Autodesk Inventor part; units mm, degrees
(part 3 of 3)
  line L1297 (279.9003, 88.0576) -> (279.8208, 87.9559)
  line L1298 (279.8208, 87.9559) -> (279.7345, 87.86)
  line L1299 (279.7345, 87.86) -> (279.6416, 87.7704)
  line L1300 (279.6416, 87.7704) -> (279.5428, 87.6874)
  line L1301 (279.5428, 87.6874) -> (279.4383, 87.6115)
  line L1302 (279.4383, 87.6115) -> (279.3289, 87.5431)
  line L1303 (279.3289, 87.5431) -> (279.2149, 87.4825)
  line L1304 (279.2149, 87.4825) -> (279.097, 87.43)
  line L1305 (279.097, 87.43) -> (278.9757, 87.3859)
  line L1306 (278.9757, 87.3859) -> (278.8517, 87.3503)
  line L1307 (278.8517, 87.3503) -> (278.7254, 87.3235)
  line L1308 (278.7254, 87.3235) -> (278.5976, 87.3055)
  line L1309 (278.5976, 87.3055) -> (278.4689, 87.2965)
  line L1310 (278.4689, 87.2965) -> (278.3398, 87.2965)
  line L1311 (278.3398, 87.2965) -> (278.211, 87.3055)
  line L1312 (278.211, 87.3055) -> (278.0832, 87.3235)
  line L1313 (278.0832, 87.3235) -> (277.957, 87.3503)
  line L1314 (277.957, 87.3503) -> (277.8329, 87.3859)
  line L1315 (277.8329, 87.3859) -> (277.7116, 87.43)
  line L1316 (277.7116, 87.43) -> (277.5937, 87.4825)
  line L1317 (277.5937, 87.4825) -> (277.4798, 87.5431)
  line L1318 (277.4798, 87.5431) -> (277.3703, 87.6115)
  line L1319 (277.3703, 87.6115) -> (277.2659, 87.6874)
  line L1320 (277.2659, 87.6874) -> (277.167, 87.7704)
  line L1321 (277.167, 87.7704) -> (277.0742, 87.86)
  line L1322 (277.0742, 87.86) -> (276.9878, 87.9559)
  line L1323 (276.9878, 87.9559) -> (276.9084, 88.0576)
  line L1324 (276.9084, 88.0576) -> (276.8362, 88.1646)
  line L1325 (276.8362, 88.1646) -> (276.7716, 88.2764)
  line L1326 (276.7716, 88.2764) -> (276.7151, 88.3924)
  line L1327 (276.7151, 88.3924) -> (276.6667, 88.5121)
  line L1328 (276.6667, 88.5121) -> (276.6268, 88.6348)
  line L1329 (276.6268, 88.6348) -> (276.5956, 88.7601)
  line L1330 (276.5956, 88.7601) -> (276.5732, 88.8872)
  line L1331 (276.5732, 88.8872) -> (276.5597, 89.0155)
  line L1332 (276.5597, 89.0155) -> (276.5552, 89.1445)
  line L1333 (276.5552, 89.1445) -> (276.5597, 89.2735)
  line L1334 (276.5597, 89.2735) -> (276.5732, 89.4019)
  line L1335 (276.5732, 89.4019) -> (276.5956, 89.529)
  line L1336 (276.5956, 89.529) -> (276.6268, 89.6542)
  line L1337 (276.6268, 89.6542) -> (276.6667, 89.777)
  line L1338 (276.6667, 89.777) -> (276.7151, 89.8966)
  line L1339 (276.7151, 89.8966) -> (276.7716, 90.0126)
  line L1340 (276.7716, 90.0126) -> (276.8362, 90.1244)
  line L1341 (276.8362, 90.1244) -> (276.9084, 90.2314)
  line L1342 (276.9084, 90.2314) -> (276.9878, 90.3331)
  line L1343 (276.9878, 90.3331) -> (277.0742, 90.429)
  line L1344 (277.0742, 90.429) -> (277.167, 90.5187)
  line L1345 (277.167, 90.5187) -> (277.2659, 90.6016)
  line L1346 (277.2659, 90.6016) -> (277.3703, 90.6775)
  line L1347 (277.3703, 90.6775) -> (277.4798, 90.7459)
  line L1348 (277.4798, 90.7459) -> (277.5937, 90.8065)
  line L1349 (277.5937, 90.8065) -> (277.7116, 90.859)
  line L1350 (277.7116, 90.859) -> (277.8329, 90.9031)
  line L1351 (277.8329, 90.9031) -> (277.957, 90.9387)
  line L1352 (277.957, 90.9387) -> (278.0832, 90.9655)
  line L1353 (278.0832, 90.9655) -> (278.211, 90.9835)
  line L1354 (278.211, 90.9835) -> (278.3398, 90.9925)
  line L1355 (278.3398, 90.9925) -> (278.4689, 90.9925)
  line L1356 (278.4689, 90.9925) -> (278.5976, 90.9835)
  line L1357 (278.5976, 90.9835) -> (278.7254, 90.9655)
  line L1358 (278.7254, 90.9655) -> (278.8517, 90.9387)
  line L1359 (278.8517, 90.9387) -> (278.9757, 90.9031)
  line L1360 (278.9757, 90.9031) -> (279.097, 90.859)
  line L1361 (279.097, 90.859) -> (279.2149, 90.8065)
  line L1362 (279.2149, 90.8065) -> (279.3289, 90.7459)
  line L1363 (279.3289, 90.7459) -> (279.4383, 90.6775)
  line L1364 (279.4383, 90.6775) -> (279.5428, 90.6016)
  line L1365 (279.5428, 90.6016) -> (279.6416, 90.5187)
  line L1366 (279.6416, 90.5187) -> (279.7345, 90.429)
  line L1367 (279.7345, 90.429) -> (279.8208, 90.3331)
  line L1368 (279.8208, 90.3331) -> (279.9003, 90.2314)
  line L1369 (279.9003, 90.2314) -> (279.9725, 90.1244)
  line L1370 (279.9725, 90.1244) -> (280.037, 90.0126)
  line L1371 (280.037, 90.0126) -> (280.0936, 89.8966)
  line L1372 (280.0936, 89.8966) -> (280.1419, 89.777)
  line L1373 (280.1419, 89.777) -> (280.1818, 89.6542)
  line L1374 (280.1818, 89.6542) -> (280.213, 89.529)
  line L1375 (280.213, 89.529) -> (280.2354, 89.4019)
  line L1376 (280.2354, 89.4019) -> (280.2489, 89.2735)
  line L1377 (280.2489, 89.2735) -> (280.2534, 89.1445)
  line L1378 (280.2534, 17.1431) -> (280.2489, 17.0142)
  line L1379 (280.2489, 17.0142) -> (280.2354, 16.8858)
  line L1380 (280.2354, 16.8858) -> (280.213, 16.7587)
  line L1381 (280.213, 16.7587) -> (280.1818, 16.6335)
  line L1382 (280.1818, 16.6335) -> (280.1419, 16.5107)
  line L1383 (280.1419, 16.5107) -> (280.0936, 16.391)
  line L1384 (280.0936, 16.391) -> (280.037, 16.275)
  line L1385 (280.037, 16.275) -> (279.9725, 16.1633)
  line L1386 (279.9725, 16.1633) -> (279.9003, 16.0563)
  line L1387 (279.9003, 16.0563) -> (279.8208, 15.9545)
  line L1388 (279.8208, 15.9545) -> (279.7345, 15.8586)
  line L1389 (279.7345, 15.8586) -> (279.6416, 15.769)
  line L1390 (279.6416, 15.769) -> (279.5428, 15.686)
  line L1391 (279.5428, 15.686) -> (279.4383, 15.6102)
  line L1392 (279.4383, 15.6102) -> (279.3289, 15.5418)
  line L1393 (279.3289, 15.5418) -> (279.2149, 15.4812)
  line L1394 (279.2149, 15.4812) -> (279.097, 15.4287)
  line L1395 (279.097, 15.4287) -> (278.9757, 15.3845)
  line L1396 (278.9757, 15.3845) -> (278.8517, 15.3489)
  line L1397 (278.8517, 15.3489) -> (278.7254, 15.3221)
  line L1398 (278.7254, 15.3221) -> (278.5976, 15.3041)
  line L1399 (278.5976, 15.3041) -> (278.4689, 15.2951)
  line L1400 (278.4689, 15.2951) -> (278.3398, 15.2951)
  line L1401 (278.3398, 15.2951) -> (278.211, 15.3041)
  line L1402 (278.211, 15.3041) -> (278.0832, 15.3221)
  line L1403 (278.0832, 15.3221) -> (277.957, 15.3489)
  line L1404 (277.957, 15.3489) -> (277.8329, 15.3845)
  line L1405 (277.8329, 15.3845) -> (277.7116, 15.4287)
  line L1406 (277.7116, 15.4287) -> (277.5937, 15.4812)
  line L1407 (277.5937, 15.4812) -> (277.4798, 15.5418)
  line L1408 (277.4798, 15.5418) -> (277.3703, 15.6102)
  line L1409 (277.3703, 15.6102) -> (277.2659, 15.686)
  line L1410 (277.2659, 15.686) -> (277.167, 15.769)
  line L1411 (277.167, 15.769) -> (277.0742, 15.8586)
  line L1412 (277.0742, 15.8586) -> (276.9878, 15.9545)
  line L1413 (276.9878, 15.9545) -> (276.9084, 16.0563)
  line L1414 (276.9084, 16.0563) -> (276.8362, 16.1633)
  line L1415 (276.8362, 16.1633) -> (276.7716, 16.275)
  line L1416 (276.7716, 16.275) -> (276.7151, 16.391)
  line L1417 (276.7151, 16.391) -> (276.6667, 16.5107)
  line L1418 (276.6667, 16.5107) -> (276.6268, 16.6335)
  line L1419 (276.6268, 16.6335) -> (276.5956, 16.7587)
  line L1420 (276.5956, 16.7587) -> (276.5732, 16.8858)
  line L1421 (276.5732, 16.8858) -> (276.5597, 17.0142)
  line L1422 (276.5597, 17.0142) -> (276.5552, 17.1431)
  line L1423 (276.5552, 17.1431) -> (276.5597, 17.2721)
  line L1424 (276.5597, 17.2721) -> (276.5732, 17.4005)
  line L1425 (276.5732, 17.4005) -> (276.5956, 17.5276)
  line L1426 (276.5956, 17.5276) -> (276.6268, 17.6528)
  line L1427 (276.6268, 17.6528) -> (276.6667, 17.7756)
  line L1428 (276.6667, 17.7756) -> (276.7151, 17.8952)
  line L1429 (276.7151, 17.8952) -> (276.7716, 18.0112)
  line L1430 (276.7716, 18.0112) -> (276.8362, 18.123)
  line L1431 (276.8362, 18.123) -> (276.9084, 18.23)
  line L1432 (276.9084, 18.23) -> (276.9878, 18.3317)
  line L1433 (276.9878, 18.3317) -> (277.0742, 18.4276)
  line L1434 (277.0742, 18.4276) -> (277.167, 18.5173)
  line L1435 (277.167, 18.5173) -> (277.2659, 18.6003)
  line L1436 (277.2659, 18.6003) -> (277.3703, 18.6761)
  line L1437 (277.3703, 18.6761) -> (277.4798, 18.7445)
  line L1438 (277.4798, 18.7445) -> (277.5937, 18.8051)
  line L1439 (277.5937, 18.8051) -> (277.7116, 18.8576)
  line L1440 (277.7116, 18.8576) -> (277.8329, 18.9018)
  line L1441 (277.8329, 18.9018) -> (277.957, 18.9373)
  line L1442 (277.957, 18.9373) -> (278.0832, 18.9642)
  line L1443 (278.0832, 18.9642) -> (278.211, 18.9821)
  line L1444 (278.211, 18.9821) -> (278.3398, 18.9911)
  line L1445 (278.3398, 18.9911) -> (278.4689, 18.9911)
  line L1446 (278.4689, 18.9911) -> (278.5976, 18.9821)
  line L1447 (278.5976, 18.9821) -> (278.7254, 18.9642)
  line L1448 (278.7254, 18.9642) -> (278.8517, 18.9373)
  line L1449 (278.8517, 18.9373) -> (278.9757, 18.9018)
  line L1450 (278.9757, 18.9018) -> (279.097, 18.8576)
  line L1451 (279.097, 18.8576) -> (279.2149, 18.8051)
  line L1452 (279.2149, 18.8051) -> (279.3289, 18.7445)
  line L1453 (279.3289, 18.7445) -> (279.4383, 18.6761)
  line L1454 (279.4383, 18.6761) -> (279.5428, 18.6003)
  line L1455 (279.5428, 18.6003) -> (279.6416, 18.5173)
  line L1456 (279.6416, 18.5173) -> (279.7345, 18.4276)
  line L1457 (279.7345, 18.4276) -> (279.8208, 18.3317)
  line L1458 (279.8208, 18.3317) -> (279.9003, 18.23)
  line L1459 (279.9003, 18.23) -> (279.9725, 18.123)
  line L1460 (279.9725, 18.123) -> (280.037, 18.0112)
  line L1461 (280.037, 18.0112) -> (280.0936, 17.8952)
  line L1462 (280.0936, 17.8952) -> (280.1419, 17.7756)
  line L1463 (280.1419, 17.7756) -> (280.1818, 17.6528)
  line L1464 (280.1818, 17.6528) -> (280.213, 17.5276)
  line L1465 (280.213, 17.5276) -> (280.2354, 17.4005)
  line L1466 (280.2354, 17.4005) -> (280.2489, 17.2721)
  line L1467 (280.2489, 17.2721) -> (280.2534, 17.1431)
  line L1468 (416.2527, 17.1431) -> (416.2482, 17.0142)
  line L1469 (416.2482, 17.0142) -> (416.2347, 16.8858)
  line L1470 (416.2347, 16.8858) -> (416.2123, 16.7587)
  line L1471 (416.2123, 16.7587) -> (416.181, 16.6335)
  line L1472 (416.181, 16.6335) -> (416.1411, 16.5107)
  line L1473 (416.1411, 16.5107) -> (416.0928, 16.391)
  line L1474 (416.0928, 16.391) -> (416.0362, 16.275)
  line L1475 (416.0362, 16.275) -> (415.9717, 16.1633)
  line L1476 (415.9717, 16.1633) -> (415.8995, 16.0563)
  line L1477 (415.8995, 16.0563) -> (415.82, 15.9545)
  line L1478 (415.82, 15.9545) -> (415.7337, 15.8586)
  line L1479 (415.7337, 15.8586) -> (415.6408, 15.769)
  line L1480 (415.6408, 15.769) -> (415.542, 15.686)
  line L1481 (415.542, 15.686) -> (415.4376, 15.6102)
  line L1482 (415.4376, 15.6102) -> (415.3281, 15.5418)
  line L1483 (415.3281, 15.5418) -> (415.2141, 15.4812)
  line L1484 (415.2141, 15.4812) -> (415.0962, 15.4287)
  line L1485 (415.0962, 15.4287) -> (414.9749, 15.3845)
  line L1486 (414.9749, 15.3845) -> (414.8509, 15.3489)
  line L1487 (414.8509, 15.3489) -> (414.7246, 15.3221)
  line L1488 (414.7246, 15.3221) -> (414.5968, 15.3041)
  line L1489 (414.5968, 15.3041) -> (414.4681, 15.2951)
  line L1490 (414.4681, 15.2951) -> (414.339, 15.2951)
  line L1491 (414.339, 15.2951) -> (414.2103, 15.3041)
  line L1492 (414.2103, 15.3041) -> (414.0824, 15.3221)
  line L1493 (414.0824, 15.3221) -> (413.9562, 15.3489)
  line L1494 (413.9562, 15.3489) -> (413.8321, 15.3845)
  line L1495 (413.8321, 15.3845) -> (413.7108, 15.4287)
  line L1496 (413.7108, 15.4287) -> (413.5929, 15.4812)
  line L1497 (413.5929, 15.4812) -> (413.479, 15.5418)
  line L1498 (413.479, 15.5418) -> (413.3695, 15.6102)
  line L1499 (413.3695, 15.6102) -> (413.2651, 15.686)
  line L1500 (413.2651, 15.686) -> (413.1662, 15.769)
  line L1501 (413.1662, 15.769) -> (413.0734, 15.8586)
  line L1502 (413.0734, 15.8586) -> (412.987, 15.9545)
  line L1503 (412.987, 15.9545) -> (412.9076, 16.0563)
  line L1504 (412.9076, 16.0563) -> (412.8354, 16.1633)
  line L1505 (412.8354, 16.1633) -> (412.7709, 16.275)
  line L1506 (412.7709, 16.275) -> (412.7143, 16.391)
  line L1507 (412.7143, 16.391) -> (412.6659, 16.5107)
  line L1508 (412.6659, 16.5107) -> (412.6261, 16.6335)
  line L1509 (412.6261, 16.6335) -> (412.5948, 16.7587)
  line L1510 (412.5948, 16.7587) -> (412.5724, 16.8858)
  line L1511 (412.5724, 16.8858) -> (412.5589, 17.0142)
  line L1512 (412.5589, 17.0142) -> (412.5544, 17.1431)
  line L1513 (412.5544, 17.1431) -> (412.5589, 17.2721)
  line L1514 (412.5589, 17.2721) -> (412.5724, 17.4005)
  line L1515 (412.5724, 17.4005) -> (412.5948, 17.5276)
  line L1516 (412.5948, 17.5276) -> (412.6261, 17.6528)
  line L1517 (412.6261, 17.6528) -> (412.6659, 17.7756)
  line L1518 (412.6659, 17.7756) -> (412.7143, 17.8952)
  line L1519 (412.7143, 17.8952) -> (412.7709, 18.0112)
  line L1520 (412.7709, 18.0112) -> (412.8354, 18.123)
  line L1521 (412.8354, 18.123) -> (412.9076, 18.23)
  line L1522 (412.9076, 18.23) -> (412.987, 18.3317)
  line L1523 (412.987, 18.3317) -> (413.0734, 18.4276)
  line L1524 (413.0734, 18.4276) -> (413.1662, 18.5173)
  line L1525 (413.1662, 18.5173) -> (413.2651, 18.6003)
  line L1526 (413.2651, 18.6003) -> (413.3695, 18.6761)
  line L1527 (413.3695, 18.6761) -> (413.479, 18.7445)
  line L1528 (413.479, 18.7445) -> (413.5929, 18.8051)
  line L1529 (413.5929, 18.8051) -> (413.7108, 18.8576)
  line L1530 (413.7108, 18.8576) -> (413.8321, 18.9018)
  line L1531 (413.8321, 18.9018) -> (413.9562, 18.9373)
  line L1532 (413.9562, 18.9373) -> (414.0824, 18.9642)
  line L1533 (414.0824, 18.9642) -> (414.2103, 18.9821)
  line L1534 (414.2103, 18.9821) -> (414.339, 18.9911)
  line L1535 (414.339, 18.9911) -> (414.4681, 18.9911)
  line L1536 (414.4681, 18.9911) -> (414.5968, 18.9821)
  line L1537 (414.5968, 18.9821) -> (414.7246, 18.9642)
  line L1538 (414.7246, 18.9642) -> (414.8509, 18.9373)
  line L1539 (414.8509, 18.9373) -> (414.9749, 18.9018)
  line L1540 (414.9749, 18.9018) -> (415.0962, 18.8576)
  line L1541 (415.0962, 18.8576) -> (415.2141, 18.8051)
  line L1542 (415.2141, 18.8051) -> (415.3281, 18.7445)
  line L1543 (415.3281, 18.7445) -> (415.4376, 18.6761)
  line L1544 (415.4376, 18.6761) -> (415.542, 18.6003)
  line L1545 (415.542, 18.6003) -> (415.6408, 18.5173)
  line L1546 (415.6408, 18.5173) -> (415.7337, 18.4276)
  line L1547 (415.7337, 18.4276) -> (415.82, 18.3317)
  line L1548 (415.82, 18.3317) -> (415.8995, 18.23)
  line L1549 (415.8995, 18.23) -> (415.9717, 18.123)
  line L1550 (415.9717, 18.123) -> (416.0362, 18.0112)
  line L1551 (416.0362, 18.0112) -> (416.0928, 17.8952)
  line L1552 (416.0928, 17.8952) -> (416.1411, 17.7756)
  line L1553 (416.1411, 17.7756) -> (416.181, 17.6528)
  line L1554 (416.181, 17.6528) -> (416.2123, 17.5276)
  line L1555 (416.2123, 17.5276) -> (416.2347, 17.4005)
  line L1556 (416.2347, 17.4005) -> (416.2482, 17.2721)
  line L1557 (416.2482, 17.2721) -> (416.2527, 17.1431)
  line L1558 (416.2527, 89.1445) -> (416.2482, 89.0155)
  line L1559 (416.2482, 89.0155) -> (416.2347, 88.8872)
  line L1560 (416.2347, 88.8872) -> (416.2123, 88.7601)
  line L1561 (416.2123, 88.7601) -> (416.181, 88.6348)
  line L1562 (416.181, 88.6348) -> (416.1411, 88.5121)
  line L1563 (416.1411, 88.5121) -> (416.0928, 88.3924)
  line L1564 (416.0928, 88.3924) -> (416.0362, 88.2764)
  line L1565 (416.0362, 88.2764) -> (415.9717, 88.1646)
  line L1566 (415.9717, 88.1646) -> (415.8995, 88.0576)
  line L1567 (415.8995, 88.0576) -> (415.82, 87.9559)
  line L1568 (415.82, 87.9559) -> (415.7337, 87.86)
  line L1569 (415.7337, 87.86) -> (415.6408, 87.7704)
  line L1570 (415.6408, 87.7704) -> (415.542, 87.6874)
  line L1571 (415.542, 87.6874) -> (415.4376, 87.6115)
  line L1572 (415.4376, 87.6115) -> (415.3281, 87.5431)
  line L1573 (415.3281, 87.5431) -> (415.2141, 87.4825)
  line L1574 (415.2141, 87.4825) -> (415.0962, 87.43)
  line L1575 (415.0962, 87.43) -> (414.9749, 87.3859)
  line L1576 (414.9749, 87.3859) -> (414.8509, 87.3503)
  line L1577 (414.8509, 87.3503) -> (414.7246, 87.3235)
  line L1578 (414.7246, 87.3235) -> (414.5968, 87.3055)
  line L1579 (414.5968, 87.3055) -> (414.4681, 87.2965)
  line L1580 (414.4681, 87.2965) -> (414.339, 87.2965)
  line L1581 (414.339, 87.2965) -> (414.2103, 87.3055)
  line L1582 (414.2103, 87.3055) -> (414.0824, 87.3235)
  line L1583 (414.0824, 87.3235) -> (413.9562, 87.3503)
  line L1584 (413.9562, 87.3503) -> (413.8321, 87.3859)
  line L1585 (413.8321, 87.3859) -> (413.7108, 87.43)
  line L1586 (413.7108, 87.43) -> (413.5929, 87.4825)
  line L1587 (413.5929, 87.4825) -> (413.479, 87.5431)
  line L1588 (413.479, 87.5431) -> (413.3695, 87.6115)
  line L1589 (413.3695, 87.6115) -> (413.2651, 87.6874)
  line L1590 (413.2651, 87.6874) -> (413.1662, 87.7704)
  line L1591 (413.1662, 87.7704) -> (413.0734, 87.86)
  line L1592 (413.0734, 87.86) -> (412.987, 87.9559)
  line L1593 (412.987, 87.9559) -> (412.9076, 88.0576)
  line L1594 (412.9076, 88.0576) -> (412.8354, 88.1646)
  line L1595 (412.8354, 88.1646) -> (412.7709, 88.2764)
  line L1596 (412.7709, 88.2764) -> (412.7143, 88.3924)
  line L1597 (412.7143, 88.3924) -> (412.6659, 88.5121)
  line L1598 (412.6659, 88.5121) -> (412.6261, 88.6348)
  line L1599 (412.6261, 88.6348) -> (412.5948, 88.7601)
  line L1600 (412.5948, 88.7601) -> (412.5724, 88.8872)
  line L1601 (412.5724, 88.8872) -> (412.5589, 89.0155)
  line L1602 (412.5589, 89.0155) -> (412.5544, 89.1445)
  line L1603 (412.5544, 89.1445) -> (412.5589, 89.2735)
  line L1604 (412.5589, 89.2735) -> (412.5724, 89.4019)
  line L1605 (412.5724, 89.4019) -> (412.5948, 89.529)
  line L1606 (412.5948, 89.529) -> (412.6261, 89.6542)
  line L1607 (412.6261, 89.6542) -> (412.6659, 89.777)
  line L1608 (412.6659, 89.777) -> (412.7143, 89.8966)
  line L1609 (412.7143, 89.8966) -> (412.7709, 90.0126)
  line L1610 (412.7709, 90.0126) -> (412.8354, 90.1244)
  line L1611 (412.8354, 90.1244) -> (412.9076, 90.2314)
  line L1612 (412.9076, 90.2314) -> (412.987, 90.3331)
  line L1613 (412.987, 90.3331) -> (413.0734, 90.429)
  line L1614 (413.0734, 90.429) -> (413.1662, 90.5187)
  line L1615 (413.1662, 90.5187) -> (413.2651, 90.6016)
  line L1616 (413.2651, 90.6016) -> (413.3695, 90.6775)
  line L1617 (413.3695, 90.6775) -> (413.479, 90.7459)
  line L1618 (413.479, 90.7459) -> (413.5929, 90.8065)
  line L1619 (413.5929, 90.8065) -> (413.7108, 90.859)
  line L1620 (413.7108, 90.859) -> (413.8321, 90.9031)
  line L1621 (413.8321, 90.9031) -> (413.9562, 90.9387)
  line L1622 (413.9562, 90.9387) -> (414.0824, 90.9655)
  line L1623 (414.0824, 90.9655) -> (414.2103, 90.9835)
  line L1624 (414.2103, 90.9835) -> (414.339, 90.9925)
  line L1625 (414.339, 90.9925) -> (414.4681, 90.9925)
  line L1626 (414.4681, 90.9925) -> (414.5968, 90.9835)
  line L1627 (414.5968, 90.9835) -> (414.7246, 90.9655)
  line L1628 (414.7246, 90.9655) -> (414.8509, 90.9387)
  line L1629 (414.8509, 90.9387) -> (414.9749, 90.9031)
  line L1630 (414.9749, 90.9031) -> (415.0962, 90.859)
  line L1631 (415.0962, 90.859) -> (415.2141, 90.8065)
  line L1632 (415.2141, 90.8065) -> (415.3281, 90.7459)
  line L1633 (415.3281, 90.7459) -> (415.4376, 90.6775)
  line L1634 (415.4376, 90.6775) -> (415.542, 90.6016)
  line L1635 (415.542, 90.6016) -> (415.6408, 90.5187)
  line L1636 (415.6408, 90.5187) -> (415.7337, 90.429)
  line L1637 (415.7337, 90.429) -> (415.82, 90.3331)
  line L1638 (415.82, 90.3331) -> (415.8995, 90.2314)
  line L1639 (415.8995, 90.2314) -> (415.9717, 90.1244)
  line L1640 (415.9717, 90.1244) -> (416.0362, 90.0126)
  line L1641 (416.0362, 90.0126) -> (416.0928, 89.8966)
  line L1642 (416.0928, 89.8966) -> (416.1411, 89.777)
  line L1643 (416.1411, 89.777) -> (416.181, 89.6542)
  line L1644 (416.181, 89.6542) -> (416.2123, 89.529)
  line L1645 (416.2123, 89.529) -> (416.2347, 89.4019)
  line L1646 (416.2347, 89.4019) -> (416.2482, 89.2735)
  line L1647 (416.2482, 89.2735) -> (416.2527, 89.1445)
  line L1648 (141.7872, 174.5398) -> (299.887, 174.5398)
  line L1649 (299.887, 174.5398) -> (299.887, 95.5407)
  line L1650 (299.887, 95.5407) -> (141.7872, 95.5407)
  line L1651 (141.7872, 95.5407) -> (141.7872, 174.5398)
  line L1652 (141.7872, 174.5398) -> (299.887, 174.5398)
  line L1653 (299.887, 174.5398) -> (299.887, 95.5407)
  line L1654 (299.887, 95.5407) -> (141.7872, 95.5407)
  line L1655 (141.7872, 95.5407) -> (141.7872, 174.5398)
  line L1656 (148.0356, 168.2584) -> (148.0311, 168.1294)
  line L1657 (148.0311, 168.1294) -> (148.0176, 168.001)
  line L1658 (148.0176, 168.001) -> (147.9952, 167.8739)
  line L1659 (147.9952, 167.8739) -> (147.964, 167.7487)
  line L1660 (147.964, 167.7487) -> (147.9241, 167.6259)
  line L1661 (147.9241, 167.6259) -> (147.8757, 167.5063)
  line L1662 (147.8757, 167.5063) -> (147.8192, 167.3903)
  line L1663 (147.8192, 167.3903) -> (147.7546, 167.2785)
  line L1664 (147.7546, 167.2785) -> (147.6824, 167.1715)
  line L1665 (147.6824, 167.1715) -> (147.603, 167.0698)
  line L1666 (147.603, 167.0698) -> (147.5166, 166.9739)
  line L1667 (147.5166, 166.9739) -> (147.4238, 166.8842)
  line L1668 (147.4238, 166.8842) -> (147.3249, 166.8012)
  line L1669 (147.3249, 166.8012) -> (147.2205, 166.7254)
  line L1670 (147.2205, 166.7254) -> (147.111, 166.657)
  line L1671 (147.111, 166.657) -> (146.9971, 166.5964)
  line L1672 (146.9971, 166.5964) -> (146.8792, 166.5439)
  line L1673 (146.8792, 166.5439) -> (146.7579, 166.4997)
  line L1674 (146.7579, 166.4997) -> (146.6338, 166.4642)
  line L1675 (146.6338, 166.4642) -> (146.5076, 166.4373)
  line L1676 (146.5076, 166.4373) -> (146.3798, 166.4194)
  line L1677 (146.3798, 166.4194) -> (146.251, 166.4104)
  line L1678 (146.251, 166.4104) -> (146.1219, 166.4104)
  line L1679 (146.1219, 166.4104) -> (145.9932, 166.4194)
  line L1680 (145.9932, 166.4194) -> (145.8654, 166.4373)
  line L1681 (145.8654, 166.4373) -> (145.7391, 166.4642)
  line L1682 (145.7391, 166.4642) -> (145.6151, 166.4997)
  line L1683 (145.6151, 166.4997) -> (145.4938, 166.5439)
  line L1684 (145.4938, 166.5439) -> (145.3759, 166.5964)
  line L1685 (145.3759, 166.5964) -> (145.2619, 166.657)
  line L1686 (145.2619, 166.657) -> (145.1525, 166.7254)
  line L1687 (145.1525, 166.7254) -> (145.048, 166.8012)
  line L1688 (145.048, 166.8012) -> (144.9492, 166.8842)
  line L1689 (144.9492, 166.8842) -> (144.8563, 166.9739)
  line L1690 (144.8563, 166.9739) -> (144.77, 167.0698)
  line L1691 (144.77, 167.0698) -> (144.6905, 167.1715)
  line L1692 (144.6905, 167.1715) -> (144.6183, 167.2785)
  line L1693 (144.6183, 167.2785) -> (144.5538, 167.3903)
  line L1694 (144.5538, 167.3903) -> (144.4972, 167.5063)
  line L1695 (144.4972, 167.5063) -> (144.4489, 167.6259)
  line L1696 (144.4489, 167.6259) -> (144.409, 167.7487)
  line L1697 (144.409, 167.7487) -> (144.3778, 167.8739)
  line L1698 (144.3778, 167.8739) -> (144.3554, 168.001)
  line L1699 (144.3554, 168.001) -> (144.3419, 168.1294)
  line L1700 (144.3419, 168.1294) -> (144.3374, 168.2584)
  line L1701 (144.3374, 168.2584) -> (144.3419, 168.3873)
  line L1702 (144.3419, 168.3873) -> (144.3554, 168.5157)
  line L1703 (144.3554, 168.5157) -> (144.3778, 168.6428)
  line L1704 (144.3778, 168.6428) -> (144.409, 168.768)
  line L1705 (144.409, 168.768) -> (144.4489, 168.8908)
  line L1706 (144.4489, 168.8908) -> (144.4972, 169.0105)
  line L1707 (144.4972, 169.0105) -> (144.5538, 169.1265)
  line L1708 (144.5538, 169.1265) -> (144.6183, 169.2382)
  line L1709 (144.6183, 169.2382) -> (144.6905, 169.3452)
  line L1710 (144.6905, 169.3452) -> (144.77, 169.447)
  line L1711 (144.77, 169.447) -> (144.8563, 169.5429)
  line L1712 (144.8563, 169.5429) -> (144.9492, 169.6325)
  line L1713 (144.9492, 169.6325) -> (145.048, 169.7155)
  line L1714 (145.048, 169.7155) -> (145.1525, 169.7913)
  line L1715 (145.1525, 169.7913) -> (145.2619, 169.8597)
  line L1716 (145.2619, 169.8597) -> (145.3759, 169.9203)
  line L1717 (145.3759, 169.9203) -> (145.4938, 169.9728)
  line L1718 (145.4938, 169.9728) -> (145.6151, 170.017)
  line L1719 (145.6151, 170.017) -> (145.7391, 170.0526)
  line L1720 (145.7391, 170.0526) -> (145.8654, 170.0794)
  line L1721 (145.8654, 170.0794) -> (145.9932, 170.0974)
  line L1722 (145.9932, 170.0974) -> (146.1219, 170.1064)
  line L1723 (146.1219, 170.1064) -> (146.251, 170.1064)
  line L1724 (146.251, 170.1064) -> (146.3798, 170.0974)
  line L1725 (146.3798, 170.0974) -> (146.5076, 170.0794)
  line L1726 (146.5076, 170.0794) -> (146.6338, 170.0526)
  line L1727 (146.6338, 170.0526) -> (146.7579, 170.017)
  line L1728 (146.7579, 170.017) -> (146.8792, 169.9728)
  line L1729 (146.8792, 169.9728) -> (146.9971, 169.9203)
  line L1730 (146.9971, 169.9203) -> (147.111, 169.8597)
  line L1731 (147.111, 169.8597) -> (147.2205, 169.7913)
  line L1732 (147.2205, 169.7913) -> (147.3249, 169.7155)
  line L1733 (147.3249, 169.7155) -> (147.4238, 169.6325)
  line L1734 (147.4238, 169.6325) -> (147.5166, 169.5429)
  line L1735 (147.5166, 169.5429) -> (147.603, 169.447)
  line L1736 (147.603, 169.447) -> (147.6824, 169.3452)
  line L1737 (147.6824, 169.3452) -> (147.7546, 169.2382)
  line L1738 (147.7546, 169.2382) -> (147.8192, 169.1265)
  line L1739 (147.8192, 169.1265) -> (147.8757, 169.0105)
  line L1740 (147.8757, 169.0105) -> (147.9241, 168.8908)
  line L1741 (147.9241, 168.8908) -> (147.964, 168.768)
  line L1742 (147.964, 168.768) -> (147.9952, 168.6428)
  line L1743 (147.9952, 168.6428) -> (148.0176, 168.5157)
  line L1744 (148.0176, 168.5157) -> (148.0311, 168.3873)
  line L1745 (148.0311, 168.3873) -> (148.0356, 168.2584)
  line L1746 (296.8034, 168.2584) -> (296.7989, 168.1294)
  line L1747 (296.7989, 168.1294) -> (296.7854, 168.001)
  line L1748 (296.7854, 168.001) -> (296.763, 167.8739)
  line L1749 (296.763, 167.8739) -> (296.7318, 167.7487)
  line L1750 (296.7318, 167.7487) -> (296.6919, 167.6259)
  line L1751 (296.6919, 167.6259) -> (296.6435, 167.5063)
  line L1752 (296.6435, 167.5063) -> (296.587, 167.3903)
  line L1753 (296.587, 167.3903) -> (296.5224, 167.2785)
  line L1754 (296.5224, 167.2785) -> (296.4502, 167.1715)
  line L1755 (296.4502, 167.1715) -> (296.3708, 167.0698)
  line L1756 (296.3708, 167.0698) -> (296.2844, 166.9739)
  line L1757 (296.2844, 166.9739) -> (296.1916, 166.8842)
  line L1758 (296.1916, 166.8842) -> (296.0927, 166.8012)
  line L1759 (296.0927, 166.8012) -> (295.9883, 166.7254)
  line L1760 (295.9883, 166.7254) -> (295.8788, 166.657)
  line L1761 (295.8788, 166.657) -> (295.7649, 166.5964)
  line L1762 (295.7649, 166.5964) -> (295.647, 166.5439)
  line L1763 (295.647, 166.5439) -> (295.5257, 166.4997)
  line L1764 (295.5257, 166.4997) -> (295.4016, 166.4642)
  line L1765 (295.4016, 166.4642) -> (295.2754, 166.4373)
  line L1766 (295.2754, 166.4373) -> (295.1476, 166.4194)
  line L1767 (295.1476, 166.4194) -> (295.0188, 166.4104)
  line L1768 (295.0188, 166.4104) -> (294.8897, 166.4104)
  line L1769 (294.8897, 166.4104) -> (294.761, 166.4194)
  line L1770 (294.761, 166.4194) -> (294.6332, 166.4373)
  line L1771 (294.6332, 166.4373) -> (294.5069, 166.4642)
  line L1772 (294.5069, 166.4642) -> (294.3829, 166.4997)
  line L1773 (294.3829, 166.4997) -> (294.2616, 166.5439)
  line L1774 (294.2616, 166.5439) -> (294.1437, 166.5964)
  line L1775 (294.1437, 166.5964) -> (294.0297, 166.657)
  line L1776 (294.0297, 166.657) -> (293.9203, 166.7254)
  line L1777 (293.9203, 166.7254) -> (293.8158, 166.8012)
  line L1778 (293.8158, 166.8012) -> (293.717, 166.8842)
  line L1779 (293.717, 166.8842) -> (293.6241, 166.9739)
  line L1780 (293.6241, 166.9739) -> (293.5378, 167.0698)
  line L1781 (293.5378, 167.0698) -> (293.4583, 167.1715)
  line L1782 (293.4583, 167.1715) -> (293.3861, 167.2785)
  line L1783 (293.3861, 167.2785) -> (293.3216, 167.3903)
  line L1784 (293.3216, 167.3903) -> (293.265, 167.5063)
  line L1785 (293.265, 167.5063) -> (293.2167, 167.6259)
  line L1786 (293.2167, 167.6259) -> (293.1768, 167.7487)
  line L1787 (293.1768, 167.7487) -> (293.1456, 167.8739)
  line L1788 (293.1456, 167.8739) -> (293.1232, 168.001)
  line L1789 (293.1232, 168.001) -> (293.1097, 168.1294)
  line L1790 (293.1097, 168.1294) -> (293.1052, 168.2584)
  line L1791 (293.1052, 168.2584) -> (293.1097, 168.3873)
  line L1792 (293.1097, 168.3873) -> (293.1232, 168.5157)
  line L1793 (293.1232, 168.5157) -> (293.1456, 168.6428)
  line L1794 (293.1456, 168.6428) -> (293.1768, 168.768)
  line L1795 (293.1768, 168.768) -> (293.2167, 168.8908)
  line L1796 (293.2167, 168.8908) -> (293.265, 169.0105)
  line L1797 (293.265, 169.0105) -> (293.3216, 169.1265)
  line L1798 (293.3216, 169.1265) -> (293.3861, 169.2382)
  line L1799 (293.3861, 169.2382) -> (293.4583, 169.3452)
  line L1800 (293.4583, 169.3452) -> (293.5378, 169.447)
  line L1801 (293.5378, 169.447) -> (293.6241, 169.5429)
  line L1802 (293.6241, 169.5429) -> (293.717, 169.6325)
  line L1803 (293.717, 169.6325) -> (293.8158, 169.7155)
  line L1804 (293.8158, 169.7155) -> (293.9203, 169.7913)
  line L1805 (293.9203, 169.7913) -> (294.0297, 169.8597)
  line L1806 (294.0297, 169.8597) -> (294.1437, 169.9203)
  line L1807 (294.1437, 169.9203) -> (294.2616, 169.9728)
  line L1808 (294.2616, 169.9728) -> (294.3829, 170.017)
  line L1809 (294.3829, 170.017) -> (294.5069, 170.0526)
  line L1810 (294.5069, 170.0526) -> (294.6332, 170.0794)
  line L1811 (294.6332, 170.0794) -> (294.761, 170.0974)
  line L1812 (294.761, 170.0974) -> (294.8897, 170.1064)
  line L1813 (294.8897, 170.1064) -> (295.0188, 170.1064)
  line L1814 (295.0188, 170.1064) -> (295.1476, 170.0974)
  line L1815 (295.1476, 170.0974) -> (295.2754, 170.0794)
  line L1816 (295.2754, 170.0794) -> (295.4016, 170.0526)
  line L1817 (295.4016, 170.0526) -> (295.5257, 170.017)
  line L1818 (295.5257, 170.017) -> (295.647, 169.9728)
  line L1819 (295.647, 169.9728) -> (295.7649, 169.9203)
  line L1820 (295.7649, 169.9203) -> (295.8788, 169.8597)
  line L1821 (295.8788, 169.8597) -> (295.9883, 169.7913)
  line L1822 (295.9883, 169.7913) -> (296.0927, 169.7155)
  line L1823 (296.0927, 169.7155) -> (296.1916, 169.6325)
  line L1824 (296.1916, 169.6325) -> (296.2844, 169.5429)
  line L1825 (296.2844, 169.5429) -> (296.3708, 169.447)
  line L1826 (296.3708, 169.447) -> (296.4502, 169.3452)
  line L1827 (296.4502, 169.3452) -> (296.5224, 169.2382)
  line L1828 (296.5224, 169.2382) -> (296.587, 169.1265)
  line L1829 (296.587, 169.1265) -> (296.6435, 169.0105)
  line L1830 (296.6435, 169.0105) -> (296.6919, 168.8908)
  line L1831 (296.6919, 168.8908) -> (296.7318, 168.768)
  line L1832 (296.7318, 168.768) -> (296.763, 168.6428)
  line L1833 (296.763, 168.6428) -> (296.7854, 168.5157)
  line L1834 (296.7854, 168.5157) -> (296.7989, 168.3873)
  line L1835 (296.7989, 168.3873) -> (296.8034, 168.2584)
  line L1836 (296.8034, 99.94) -> (296.7989, 99.811)
  line L1837 (296.7989, 99.811) -> (296.7854, 99.6826)
  line L1838 (296.7854, 99.6826) -> (296.763, 99.5555)
  line L1839 (296.763, 99.5555) -> (296.7318, 99.4303)
  line L1840 (296.7318, 99.4303) -> (296.6919, 99.3075)
  line L1841 (296.6919, 99.3075) -> (296.6435, 99.1879)
  line L1842 (296.6435, 99.1879) -> (296.587, 99.0719)
  line L1843 (296.587, 99.0719) -> (296.5224, 98.9601)
  line L1844 (296.5224, 98.9601) -> (296.4502, 98.8531)
  line L1845 (296.4502, 98.8531) -> (296.3708, 98.7514)
  line L1846 (296.3708, 98.7514) -> (296.2844, 98.6555)
  line L1847 (296.2844, 98.6555) -> (296.1916, 98.5658)
  line L1848 (296.1916, 98.5658) -> (296.0927, 98.4829)
  line L1849 (296.0927, 98.4829) -> (295.9883, 98.407)
  line L1850 (295.9883, 98.407) -> (295.8788, 98.3386)
  line L1851 (295.8788, 98.3386) -> (295.7649, 98.278)
  line L1852 (295.7649, 98.278) -> (295.647, 98.2255)
  line L1853 (295.647, 98.2255) -> (295.5257, 98.1814)
  line L1854 (295.5257, 98.1814) -> (295.4016, 98.1458)
  line L1855 (295.4016, 98.1458) -> (295.2754, 98.119)
  line L1856 (295.2754, 98.119) -> (295.1476, 98.101)
  line L1857 (295.1476, 98.101) -> (295.0188, 98.092)
  line L1858 (295.0188, 98.092) -> (294.8897, 98.092)
  line L1859 (294.8897, 98.092) -> (294.761, 98.101)
  line L1860 (294.761, 98.101) -> (294.6332, 98.119)
  line L1861 (294.6332, 98.119) -> (294.5069, 98.1458)
  line L1862 (294.5069, 98.1458) -> (294.3829, 98.1814)
  line L1863 (294.3829, 98.1814) -> (294.2616, 98.2255)
  line L1864 (294.2616, 98.2255) -> (294.1437, 98.278)
  line L1865 (294.1437, 98.278) -> (294.0297, 98.3386)
  line L1866 (294.0297, 98.3386) -> (293.9203, 98.407)
  line L1867 (293.9203, 98.407) -> (293.8158, 98.4829)
  line L1868 (293.8158, 98.4829) -> (293.717, 98.5658)
  line L1869 (293.717, 98.5658) -> (293.6241, 98.6555)
  line L1870 (293.6241, 98.6555) -> (293.5378, 98.7514)
  line L1871 (293.5378, 98.7514) -> (293.4583, 98.8531)
  line L1872 (293.4583, 98.8531) -> (293.3861, 98.9601)
  line L1873 (293.3861, 98.9601) -> (293.3216, 99.0719)
  line L1874 (293.3216, 99.0719) -> (293.265, 99.1879)
  line L1875 (293.265, 99.1879) -> (293.2167, 99.3075)
  line L1876 (293.2167, 99.3075) -> (293.1768, 99.4303)
  line L1877 (293.1768, 99.4303) -> (293.1456, 99.5555)
  line L1878 (293.1456, 99.5555) -> (293.1232, 99.6826)
  line L1879 (293.1232, 99.6826) -> (293.1097, 99.811)
  line L1880 (293.1097, 99.811) -> (293.1052, 99.94)
  line L1881 (293.1052, 99.94) -> (293.1097, 100.069)
  line L1882 (293.1097, 100.069) -> (293.1232, 100.1973)
  line L1883 (293.1232, 100.1973) -> (293.1456, 100.3244)
  line L1884 (293.1456, 100.3244) -> (293.1768, 100.4497)
  line L1885 (293.1768, 100.4497) -> (293.2167, 100.5724)
  line L1886 (293.2167, 100.5724) -> (293.265, 100.6921)
  line L1887 (293.265, 100.6921) -> (293.3216, 100.8081)
  line L1888 (293.3216, 100.8081) -> (293.3861, 100.9199)
  line L1889 (293.3861, 100.9199) -> (293.4583, 101.0269)
  line L1890 (293.4583, 101.0269) -> (293.5378, 101.1286)
  line L1891 (293.5378, 101.1286) -> (293.6241, 101.2245)
  line L1892 (293.6241, 101.2245) -> (293.717, 101.3141)
  line L1893 (293.717, 101.3141) -> (293.8158, 101.3971)
  line L1894 (293.8158, 101.3971) -> (293.9203, 101.473)
  line L1895 (293.9203, 101.473) -> (294.0297, 101.5414)
  line L1896 (294.0297, 101.5414) -> (294.1437, 101.602)
  line L1897 (294.1437, 101.602) -> (294.2616, 101.6545)
  line L1898 (294.2616, 101.6545) -> (294.3829, 101.6986)
  line L1899 (294.3829, 101.6986) -> (294.5069, 101.7342)
  line L1900 (294.5069, 101.7342) -> (294.6332, 101.761)
  line L1901 (294.6332, 101.761) -> (294.761, 101.779)
  line L1902 (294.761, 101.779) -> (294.8897, 101.788)
  line L1903 (294.8897, 101.788) -> (295.0188, 101.788)
  line L1904 (295.0188, 101.788) -> (295.1476, 101.779)
  line L1905 (295.1476, 101.779) -> (295.2754, 101.761)
  line L1906 (295.2754, 101.761) -> (295.4016, 101.7342)
  line L1907 (295.4016, 101.7342) -> (295.5257, 101.6986)
  line L1908 (295.5257, 101.6986) -> (295.647, 101.6545)
  line L1909 (295.647, 101.6545) -> (295.7649, 101.602)
  line L1910 (295.7649, 101.602) -> (295.8788, 101.5414)
  line L1911 (295.8788, 101.5414) -> (295.9883, 101.473)
  line L1912 (295.9883, 101.473) -> (296.0927, 101.3971)
  line L1913 (296.0927, 101.3971) -> (296.1916, 101.3141)
  line L1914 (296.1916, 101.3141) -> (296.2844, 101.2245)
  line L1915 (296.2844, 101.2245) -> (296.3708, 101.1286)
  line L1916 (296.3708, 101.1286) -> (296.4502, 101.0269)
  line L1917 (296.4502, 101.0269) -> (296.5224, 100.9199)
  line L1918 (296.5224, 100.9199) -> (296.587, 100.8081)
  line L1919 (296.587, 100.8081) -> (296.6435, 100.6921)
  line L1920 (296.6435, 100.6921) -> (296.6919, 100.5724)
  line L1921 (296.6919, 100.5724) -> (296.7318, 100.4497)
  line L1922 (296.7318, 100.4497) -> (296.763, 100.3244)
  line L1923 (296.763, 100.3244) -> (296.7854, 100.1973)
  line L1924 (296.7854, 100.1973) -> (296.7989, 100.069)
  line L1925 (296.7989, 100.069) -> (296.8034, 99.94)
  line L1926 (148.0356, 99.94) -> (148.0311, 99.811)
  line L1927 (148.0311, 99.811) -> (148.0176, 99.6826)
  line L1928 (148.0176, 99.6826) -> (147.9952, 99.5555)
  line L1929 (147.9952, 99.5555) -> (147.964, 99.4303)
  line L1930 (147.964, 99.4303) -> (147.9241, 99.3075)
  line L1931 (147.9241, 99.3075) -> (147.8757, 99.1879)
  line L1932 (147.8757, 99.1879) -> (147.8192, 99.0719)
  line L1933 (147.8192, 99.0719) -> (147.7546, 98.9601)
  line L1934 (147.7546, 98.9601) -> (147.6824, 98.8531)
  line L1935 (147.6824, 98.8531) -> (147.603, 98.7514)
  line L1936 (147.603, 98.7514) -> (147.5166, 98.6555)
  line L1937 (147.5166, 98.6555) -> (147.4238, 98.5658)
  line L1938 (147.4238, 98.5658) -> (147.3249, 98.4829)
  line L1939 (147.3249, 98.4829) -> (147.2205, 98.407)
  line L1940 (147.2205, 98.407) -> (147.111, 98.3386)
  line L1941 (147.111, 98.3386) -> (146.9971, 98.278)
  line L1942 (146.9971, 98.278) -> (146.8792, 98.2255)
  line L1943 (146.8792, 98.2255) -> (146.7579, 98.1814)
  line L1944 (146.7579, 98.1814) -> (146.6338, 98.1458)
  line L1945 (146.6338, 98.1458) -> (146.5076, 98.119)
  line L1946 (146.5076, 98.119) -> (146.3798, 98.101)
  line L1947 (146.3798, 98.101) -> (146.251, 98.092)
  line L1948 (146.251, 98.092) -> (146.1219, 98.092)
  line L1949 (146.1219, 98.092) -> (145.9932, 98.101)
  line L1950 (145.9932, 98.101) -> (145.8654, 98.119)
  line L1951 (145.8654, 98.119) -> (145.7391, 98.1458)
  line L1952 (145.7391, 98.1458) -> (145.6151, 98.1814)
  line L1953 (145.6151, 98.1814) -> (145.4938, 98.2255)
  line L1954 (145.4938, 98.2255) -> (145.3759, 98.278)
  line L1955 (145.3759, 98.278) -> (145.2619, 98.3386)
  line L1956 (145.2619, 98.3386) -> (145.1525, 98.407)
  line L1957 (145.1525, 98.407) -> (145.048, 98.4829)
  line L1958 (145.048, 98.4829) -> (144.9492, 98.5658)
  line L1959 (144.9492, 98.5658) -> (144.8563, 98.6555)
  line L1960 (144.8563, 98.6555) -> (144.77, 98.7514)
  line L1961 (144.77, 98.7514) -> (144.6905, 98.8531)
  line L1962 (144.6905, 98.8531) -> (144.6183, 98.9601)
  line L1963 (144.6183, 98.9601) -> (144.5538, 99.0719)
  line L1964 (144.5538, 99.0719) -> (144.4972, 99.1879)
  line L1965 (144.4972, 99.1879) -> (144.4489, 99.3075)
  line L1966 (144.4489, 99.3075) -> (144.409, 99.4303)
  line L1967 (144.409, 99.4303) -> (144.3778, 99.5555)
  line L1968 (144.3778, 99.5555) -> (144.3554, 99.6826)
  line L1969 (144.3554, 99.6826) -> (144.3419, 99.811)
  line L1970 (144.3419, 99.811) -> (144.3374, 99.94)
  line L1971 (144.3374, 99.94) -> (144.3419, 100.069)
  line L1972 (144.3419, 100.069) -> (144.3554, 100.1973)
  line L1973 (144.3554, 100.1973) -> (144.3778, 100.3244)
  line L1974 (144.3778, 100.3244) -> (144.409, 100.4497)
  line L1975 (144.409, 100.4497) -> (144.4489, 100.5724)
  line L1976 (144.4489, 100.5724) -> (144.4972, 100.6921)
  line L1977 (144.4972, 100.6921) -> (144.5538, 100.8081)
  line L1978 (144.5538, 100.8081) -> (144.6183, 100.9199)
  line L1979 (144.6183, 100.9199) -> (144.6905, 101.0269)
  line L1980 (144.6905, 101.0269) -> (144.77, 101.1286)
  line L1981 (144.77, 101.1286) -> (144.8563, 101.2245)
  line L1982 (144.8563, 101.2245) -> (144.9492, 101.3141)
  line L1983 (144.9492, 101.3141) -> (145.048, 101.3971)
  line L1984 (145.048, 101.3971) -> (145.1525, 101.473)
  line L1985 (145.1525, 101.473) -> (145.2619, 101.5414)
  line L1986 (145.2619, 101.5414) -> (145.3759, 101.602)
  line L1987 (145.3759, 101.602) -> (145.4938, 101.6545)
  line L1988 (145.4938, 101.6545) -> (145.6151, 101.6986)
  line L1989 (145.6151, 101.6986) -> (145.7391, 101.7342)
  line L1990 (145.7391, 101.7342) -> (145.8654, 101.761)
  line L1991 (145.8654, 101.761) -> (145.9932, 101.779)
  line L1992 (145.9932, 101.779) -> (146.1219, 101.788)
  line L1993 (146.1219, 101.788) -> (146.251, 101.788)
  line L1994 (146.251, 101.788) -> (146.3798, 101.779)
  line L1995 (146.3798, 101.779) -> (146.5076, 101.761)
  line L1996 (146.5076, 101.761) -> (146.6338, 101.7342)
  line L1997 (146.6338, 101.7342) -> (146.7579, 101.6986)
  line L1998 (146.7579, 101.6986) -> (146.8792, 101.6545)
  line L1999 (146.8792, 101.6545) -> (146.9971, 101.602)
  line L2000 (146.9971, 101.602) -> (147.111, 101.5414)
  line L2001 (147.111, 101.5414) -> (147.2205, 101.473)
  line L2002 (147.2205, 101.473) -> (147.3249, 101.3971)
  line L2003 (147.3249, 101.3971) -> (147.4238, 101.3141)
  line L2004 (147.4238, 101.3141) -> (147.5166, 101.2245)
  line L2005 (147.5166, 101.2245) -> (147.603, 101.1286)
  line L2006 (147.603, 101.1286) -> (147.6824, 101.0269)
  line L2007 (147.6824, 101.0269) -> (147.7546, 100.9199)
  line L2008 (147.7546, 100.9199) -> (147.8192, 100.8081)
  line L2009 (147.8192, 100.8081) -> (147.8757, 100.6921)
  line L2010 (147.8757, 100.6921) -> (147.9241, 100.5724)
  line L2011 (147.9241, 100.5724) -> (147.964, 100.4497)
  line L2012 (147.964, 100.4497) -> (147.9952, 100.3244)
  line L2013 (147.9952, 100.3244) -> (148.0176, 100.1973)
  line L2014 (148.0176, 100.1973) -> (148.0311, 100.069)
  line L2015 (148.0311, 100.069) -> (148.0356, 99.94)
  point P0 (0, 0)
  constraints: 4032 end point
extrude "Cut4" cut sketch "Sketch2" against normal blind 3.175 contours A0 | L0 A1 L1 A2 | L2 A3 L3 A4 | L4 A5 L5 A6 | L6 A7 L7 A8 | L8 A9 L9 A10 | L10 A11 L11 A12 | L12 A13 L13 A14 | A18 L17 A17 L16 A16 L15 A15 L14 | A26 L25 A25 L24 A24 L23 A23 L22 | A34 L33 A33 L32 A32 L31 A31 L30 | A42 L41 A41 L40 A40 L39 A39 L38 | A47 | A48 | A49 | A50 | A52 | A53 | A54 | A55 | A56 | A57 | A58 | A59 | A60 | A70 | A71 | A72 | A73 | A74 | A75 | A76 | A77 | A78 | A79 | A80 | A81 | A82 | A83 | A89 | A90 | A91 | A92 | A96 | A97 | A98 | A99 | A100 | A101 | A102 | A103 | A104 | A111 | A112 | A113 | A114 | L46 A119 L47 A120 L48 A121 L49 A118 | L50 A122 L51 A123 | L52 A124 L53 A125 | L54 A126 L55 A127 | A128 | A129 | L57 A136 L56 A135 | A165 | A166 | A167 | A168 | A185
equation "\"d7\" = MinimumRemnant"
equation "\"GapSize\" = Thickness"
equation "\"d27\" = Thickness"
equation "\"d49\" = Thickness"
equation "\"d2\" = Thickness"
equation "\"d5\" = BendReliefWidth"
equation "\"d6\" = BendReliefDepth"
equation "\"d8\" = TransitionRadius"
equation "\"d11\" = BendRadius"
equation "\"d12\" = CornerReliefSize"
equation "\"d13\" = GapSize"
equation "\"d14\" = JacobiRadiusSize"
equation "\"d17\" = BendReliefWidth"
equation "\"d18\" = BendReliefDepth"
equation "\"d19\" = MinimumRemnant"
equation "\"d20\" = TransitionRadius"
equation "\"d23\" = BendRadius"
equation "\"d24\" = CornerReliefSize"
equation "\"d25\" = GapSize"
equation "\"d26\" = JacobiRadiusSize"
equation "\"d29\" = BendReliefWidth"
equation "\"d30\" = BendReliefDepth"
equation "\"d31\" = MinimumRemnant"
equation "\"d32\" = TransitionRadius"
equation "\"d35\" = BendRadius"
equation "\"d36\" = CornerReliefSize"
equation "\"d37\" = GapSize"
equation "\"d38\" = JacobiRadiusSize"
equation "\"d39\" = BendReliefWidth"
equation "\"d40\" = BendReliefDepth"
equation "\"d41\" = MinimumRemnant"
equation "\"d42\" = TransitionRadius"
equation "\"d45\" = BendRadius"
equation "\"d46\" = CornerReliefSize"
equation "\"d47\" = GapSize"
equation "\"d48\" = JacobiRadiusSize"
equation "\"BendRadius\" = Thickness"
equation "\"BendReliefWidth\" = Thickness"
equation "\"BendReliefDepth\" = 0.5 * Thickness"
equation "\"CornerReliefSize\" = 4 * Thickness"
equation "\"MinimumRemnant\" = 2 * Thickness"
equation "\"TransitionRadius\" = BendRadius"
equation "\"JacobiRadiusSize\" = BendRadius"
equation "\"Thickness\" = 3.175"
body "Solid1"
